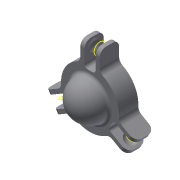
# Autodesk Inventor part: Shuttle
Saved by Autodesk Inventor 2022 Beta2 (Build 260130000, 130) ContinuousBuild 0
## iProperties
Created: 2013-03-11
Part Number: Shuttle
Material: Generic
Document SubType Name: Modeling
Designer: user
Density: 1 g/cm^3
Appearance: Default
Author: user
Autodesk Inventor part; units mm, degrees
ref_plane "XZ Plane" through (0, 0, 0) normal (0, 1, 0) x (-1, 0, 0)
ref_plane "XY Plane" through (0, 0, 0) normal (0, 0, 1) x (1, 0, 0)
sketch "Sketch1" plane through (0, 0, 0) normal (0, 0, 1) x (1, 0, 0)
  circle A0 centre (0, 0) radius 57.023
  dimension "d0" = 57.023
  constraints: 1 centre point, 1 coincident
  measures "d0" radius of A0
extrude "Extrusion1" add sketch "Sketch1" along normal mid plane 38.1
sketch "Sketch2" plane through (0, 0, 0) normal (0, 0, 1) x (1, 0, 0)
  circle A0 centre (0, 0) radius 57.023
  line L0 (0, 0) -> (0, 76.2) construction
  circle A1 centre (0, 76.2) radius 15.875
  line L1 (-19.05, 92.075) -> (19.05, 92.075)
  line L2 (19.05, 92.075) -> (19.05, 47.625)
  line L3 (19.05, 47.625) -> (-19.05, 47.625)
  line L4 (-19.05, 47.625) -> (-19.05, 92.075)
  line L5 (-11.1125, 92.075) -> (11.1125, 92.075)
  line L6 (11.1125, 92.075) -> (11.1125, 47.625)
  line L7 (11.1125, 47.625) -> (-11.1125, 47.625)
  line L8 (-11.1125, 47.625) -> (-11.1125, 92.075)
  line L9 (0, 92.075) -> (0, 60.325)
  point P0 (0, 47.625)
  point P1 (0, 47.625)
  dimension "d4" = 15.875
  dimension "d6" = 76.2
  dimension "d7" = 15.875
  dimension "d8" = 19.05
  dimension "d9" = 47.625
  dimension "d10" = 22.225
  constraints: 20 end point, 4 parallel, 3 point on line, 2 centre point, 2 collinear, 2 horizontal, 2 midpoint, 2 perpendicular, 2 point on circle, 1 coincident, 1 vertical
  measures "d4" radius of A1
  measures "d6" distance of L0.start L0.end
  measures "d7" distance from line of A1.centre L1
  measures "d8" distance from line of A1.centre L4
  measures "d9" distance from line of L0.start L3
  measures "d10" distance between parallel lines of L6 L8
extrude "Extrusion2" add sketch "Sketch2" against normal up to surface (38.1 mm away) from surface at 19.05 contours L2 L3 L6 A0 | A0 L6 A1 L1 L2 | L4 L1 L8 A1 A0 | A0 L8 L3 L4 | L6 L3 L8 A0 | A0 L8 A1 L6 | L6 A1 | A1 L9 L6 | L6 A1 L1 | L8 A1 L9 | A1 L8 | L1 A1 L8
extrude "Extrusion3" cut sketch "Sketch2" along normal through all both and the other way through all contours L6 L3 L8 A0 | A0 L8 A1 L6 | A1 L9 L6 | L6 A1 L1 | L8 A1 L9 | L1 A1 L8
revolve "Revolution1" cut sketch "Sketch2" angle 360 about axis through (0, 92.075, 0) along (0, -1, 0) contours L8 A1 L9 | A1 L8
fillet "Fillet1" radius 12.7 6 edges at (-15.0813, 92.075, 19.05) (-15.0813, 92.075, -19.05) (15.0813, 92.075, 19.05) (15.0813, 92.075, -19.05) (19.05, 53.7468, 0) (-19.05, 53.7468, 0)
fillet "Fillet2" radius 6.35 2 edges at (-11.1125, 47.625, 0) (11.1125, 47.625, 0)
ref_plane "Work Plane2" through (0, 0, 0) normal (1, 0, 0) x (0, 0, 1)
pattern_circular "Circular Pattern1" count 3 over 360 about axis through (0, 0, 0) along (0, 0, 1) of "Extrusion2", "Extrusion3", "Revolution1", "Fillet1", "Fillet2"
sketch "Ball Joint Ref1" plane through (0, 0, 0) normal (1, 0, 0) x (0, 0, 1)
  circle A0 centre (0, -76.2) radius 11.337 projected
  point P0 (0, 0)
sketch "Ball Joint Ref2" plane through (0, 0, 0) normal (-0.5, -0.8660254, 0) x (0, 0, 1)
  circle A0 centre (0, -76.2) radius 11.337 projected
  point P0 (0, 0)
sketch "Ball Joint Ref3" plane through (0, 0, 0) normal (-0.5, 0.8660254, 0) x (0, 0, 1)
  circle A0 centre (0, -76.2) radius 11.337 projected
  point P0 (0, 0)
sketch "Sketch3" plane through (0, 0, 19.05) normal (0, 0, 1) x (1, 0, 0)
  line L0 (-19.05, 62.0744) -> (-19.05, 79.375) projected
  arc A0 (-30.9827, -47.8717) -> (30.9827, -47.8717) centre (0, 0) ccw projected
  circle A1 centre (0, 0) radius 38.1
  line L1 (0, 38.1) -> (0, -38.1)
  dimension "d21" = 76.2
  constraints: 2 end point, 2 point on circle, 1 centre point, 1 coincident, 1 parallel
  measures "d21" diameter of A1
revolve "Revolution2" add sketch "Sketch3" angle 360 about axis through (0, 38.1, 19.05) along (0, -1, 0) picked at (13.4286, -11.187) contours A1 L1
fillet "Fillet3" radius 6.35 2 edges at (38.1, 0, 19.05) (-38.1, 0, 19.05)
ref_plane "Work Plane3" through (0, 0, 0) normal (-0.5, 0.8660254, 0) x (0, 0, 1)
ref_plane "Work Plane4" through (0, 0, 0) normal (-0.5, -0.8660254, 0) x (0, 0, 1)
body "Solid1"
